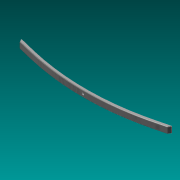
# Autodesk Inventor part: leaf 33
Saved by Autodesk Inventor 2014 SP2 (Build 180246200, 246)
## iProperties
Created: 2019-07-17
Part Number: leaf 33
Material: Steel, Carbon
Document SubType Name: Modeling
Designer: USER PC
Density: 7.87 g/cm^3
Appearance: Semi-Polished
Mass: 1961.93 g
Surface Area: 491.969 cm^2
Volume: 249.292 cm^3
Author: USER PC
Autodesk Inventor part; units mm, degrees
ref_plane "YZ Plane" through (0, 0, 0) normal (1, 0, 0) x (0, 1, 0)
ref_plane "XZ Plane" through (0, 0, 0) normal (0, 1, 0) x (-1, 0, 0)
ref_plane "XY Plane" through (0, 0, 0) normal (0, 0, 1) x (1, 0, 0)
sketch "Sketch1" plane through (0, 0, 0) normal (0, 0, 1) x (1, 0, 0)
  arc A0 (0.2695, -91.5776) -> (286.8271, -56.8995) centre (0.2695, 1109.728) ccw
  arc A1 (0.2695, -106.5776) -> (290.4052, -71.4665) centre (0.2695, 1109.728) ccw
  line L0 (0.2695, -106.5776) -> (0.2695, -82.8765)
  line L1 (0, 0) -> (363.543, 0)
  line L2 (286.8271, -56.8995) -> (363.543, -38.0559)
  line L3 (290.4052, -71.4665) -> (353.1517, -56.0541)
  line L4 (363.543, -38.0559) -> (353.1517, -56.0541)
  arc A2 (-286.2882, -56.8995) -> (0.2695, -91.5776) centre (0.2695, 1109.728) ccw
  arc A3 (-289.8663, -71.4665) -> (0.2695, -106.5776) centre (0.2695, 1109.728) ccw
  line L5 (-286.2882, -56.8995) -> (-363.0041, -38.0559)
  line L6 (-289.8663, -71.4665) -> (-352.6128, -56.0541)
  line L7 (-363.0041, -38.0559) -> (-352.6128, -56.0541)
  point P0 (254.9341, -79.6185)
  dimension "d0" = 15
  dimension "d9" = 363.543
  constraints: 16 end point, 9 point on circle, 4 centre point, 4 symmetric about line, 2 tangent, 1 parallel, 1 perpendicular, 2 other
  measures "d0" radial gap between concentric circles of A1 A0
  measures "d9" distance of L1.start L1.end
extrude "Extrusion1" add sketch "Sketch1" along normal blind 30
sketch "Sketch2" plane through (0, 0, 0) normal (0, 1, 0) x (-1, 0, 0)
  line L0 (0, 0) -> (0, 15)
  circle A0 centre (0, 15) radius 5
  dimension "d5" = 15
  dimension "d6" = 10
  constraints: 2 end point, 1 centre point, 1 coincident, 1 vertical
  measures "d5" distance of L0.start L0.end
  measures "d6" diameter of A0
extrude "Extrusion2" cut sketch "Sketch2" against normal blind 300
fillet "Fillet2" radius 3 20 edges at (-363.0041, -38.0559, 15) (-357.8084, -47.055, 0) (-357.8084, -47.055, 30) (-352.6128, -56.0541, 15) (146.3957, -97.7679, 30) (321.7784, -63.7603, 30) (-321.2395, -63.7603, 30) (146.3957, -97.7679, 0) (321.7784, -63.7603, 0) (-321.2395, -63.7603, 0) (-144.0547, -82.8765, 30) (325.1851, -47.4777, 30) (-324.6461, -47.4777, 30) (358.3473, -47.055, 30) (363.543, -38.0559, 15) (144.5936, -82.8765, 0) (-324.6461, -47.4777, 0) (325.1851, -47.4777, 0) (358.3473, -47.055, 0) (353.1517, -56.0541, 15)
body "Solid1"
